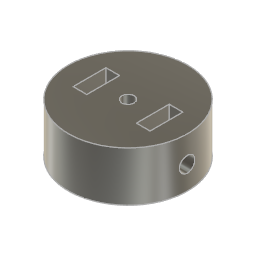
coupling gear v9 (Autodesk Fusion 360 design; units mm, degrees)
Autodesk Fusion 360 part; units mm, degrees
sketch "Sketch1" plane through (0, 0, 0) normal (0, 0, 1) x (1, 0, 0)
  circle A0 centre (0, 0) radius 12
  circle A1 centre (0, 0) radius 1.25
  dimension "d1" = 2.5
  dimension "d12" = 24
  constraint coincident A0.centre A1.centre
  measures "d1" diameter of A1
  measures "d12" diameter of A0
extrude "Extrude1" add sketch "Sketch1" along normal blind 10
sketch "Sketch2" plane through (0, 0, 0) normal (1, 0, 0) x (0, 1, 0)
  circle A0 centre (0, 4.686) radius 1.55
  dimension "d4" = 3.1
  measures "d4" diameter of A0
extrude "Extrude2" cut sketch "Sketch2" along normal blind 12 and the other way blind 12
sketch "Sketch3" plane through (0, 0, 10) normal (0, 0, 1) x (-1, 0, 0)
  circle A0 centre (0, 0) radius 1.25
  circle A1 centre (0, 0) radius 12
  line L0 (-5, 0.003) -> (-5, 3.303)
  line L1 (-5, 0.003) -> (-5, -3.297)
  line L2 (-5, 3.303) -> (-7.75, 3.303)
  line L3 (-5, -3.297) -> (-7.75, -3.297)
  line L4 (-7.75, 3.303) -> (-7.75, -3.297)
  line L5 (0, -1.25) -> (0, -1.55)
  line L6 (5, 3.303) -> (7.75, 3.303)
  line L7 (5, 0.003) -> (5, 3.303)
  line L8 (5, 0.003) -> (5, -3.297)
  line L9 (7.75, 3.303) -> (7.75, -3.297)
  line L10 (5, -3.297) -> (7.75, -3.297)
  dimension "d7" = 3.3
  dimension "d8" = 3.3
  dimension "d9" = 2.75
  dimension "d10" = 2.75
  dimension "d11" = 5
  constraint vertical L0
  constraint parallel L0 L1
  constraint perpendicular L0 L2
  constraint perpendicular L1 L3
  constraint symmetric L0.start L5 L7.start
  constraint symmetric L0.end L5 L6.start
  constraint symmetric L1.end L5 L8.end
  constraint symmetric L2.end L5 L6.end
  constraint symmetric L3.end L5 L9.end
  measures "d7" distance of L0.start L0.end
  measures "d8" distance of L0.start L1.end
  measures "d9" distance of L0.end L2.end
  measures "d10" distance of L1.end L3.end
  measures "d11" distance of A0.centre L0
extrude "Extrude4" cut sketch "Sketch3" against normal blind 8 contours L0 L1 L2 L3 L4 | L6 L7 L8 L9 L10
